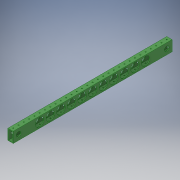
# Autodesk Inventor part: Kermit Frame 14
Saved by Autodesk Inventor 2018.2 (Build 222227000, 227)
## iProperties
Created: 2018-02-17
Part Number: Kermit Frame 14
Material: Generic
Document SubType Name: Modeling
Designer: lopez.xavier
Density: 1 g/cm^3
Appearance: Smooth - Dark Forest Green
Author: lopez.xavier
Autodesk Inventor part; units mm, degrees
ref_plane "YZ Plane" through (0, 0, 0) normal (1, 0, 0) x (0, 1, 0)
ref_plane "XZ Plane" through (0, 0, 0) normal (0, 1, 0) x (-1, 0, 0)
ref_plane "XY Plane" through (0, 0, 0) normal (0, 0, 1) x (1, 0, 0)
sketch "Sketch1" plane through (0, 0, 0) normal (0, 0, 1) x (1, 0, 0)
  line L0 (0, 0) -> (25.4, 0)
  line L1 (25.4, 0) -> (25.4, 50.8)
  line L2 (25.4, 50.8) -> (0, 50.8)
  line L3 (0, 50.8) -> (0, 0)
  dimension "d0" = 50.8
  dimension "d1" = 25.4
  constraints: 8 end point, 2 parallel, 1 horizontal, 1 perpendicular
  measures "d0" distance of L0.end L1.end
  measures "d1" distance of L1.end L2.end
extrude "Extrusion1" add sketch "Sketch1" along normal blind 762
shell "Shell1" thickness 3.175 removed faces 2 at (16.9333, 16.9333, 0) at (16.9333, 16.9333, 762)
sketch "Sketch2" plane through (25.4, 0, 0) normal (1, 0, 0) x (0, 0, -1)
  circle A0 centre (-635, 25.4) radius 20.32
  line L0 (0, 50.8) -> (-762, 50.8) projected
  circle A1 centre (-584.2, 25.4) radius 20.32
  circle A2 centre (-533.4, 25.4) radius 20.32
  circle A3 centre (-482.6, 25.4) radius 20.32
  circle A4 centre (-431.8, 25.4) radius 20.32
  circle A5 centre (-381, 25.4) radius 20.32
  circle A6 centre (-330.2, 25.4) radius 20.32
  circle A7 centre (-279.4, 25.4) radius 20.32
  circle A8 centre (-228.6, 25.4) radius 20.32
  circle A9 centre (-177.8, 25.4) radius 20.32
  circle A10 centre (-127, 25.4) radius 20.32
  line L1 (-762, 0) -> (-762, 50.8) projected
  circle A11 centre (-736.6, 25.4) radius 11.43
  circle A12 centre (-25.4, 25.4) radius 11.43
  line L2 (0, 0) -> (0, 50.8) projected
  dimension "d5" = 40.64
  dimension "d6" = 25.4
  dimension "d9" = 50.8
  dimension "d14" = 127
  dimension "d17" = 22.86
  dimension "d18" = 22.86
  dimension "d19" = 25.4
  dimension "d20" = 25.4
  dimension "d21" = 25.4
  dimension "d22" = 25.4
  constraints: 13 centre point, 1 horizontal, 20 other
  measures "d5" diameter of A0
  measures "d6" distance from line of L0 A0.centre
  measures "d9" distance of A0.centre A1.centre
  measures "d14" distance from line of L1 A0.centre
  measures "d17" diameter of A11
  measures "d18" diameter of A12
  measures "d19" distance from line of L0 A11.centre
  measures "d20" distance from line of L0 A12.centre
  measures "d21" distance from line of L1 A11.centre
  measures "d22" distance from line of L2 A12.centre
extrude "Extrusion2" cut sketch "Sketch2" against normal blind 25.4
sketch "Sketch3" plane through (0, 50.8, 0) normal (0, 1, 0) x (1, 0, 0)
  circle A0 centre (12.7, -749.3) radius 2.54
  line L0 (0, 0) -> (0, -762) projected
  line L1 (25.4, -762) -> (0, -762) projected
  circle A1 centre (12.7, -723.9) radius 2.54
  circle A2 centre (12.7, -698.5) radius 2.54
  circle A3 centre (12.7, -673.1) radius 2.54
  circle A4 centre (12.7, -647.7) radius 2.54
  circle A5 centre (12.7, -622.3) radius 2.54
  circle A6 centre (12.7, -596.9) radius 2.54
  circle A7 centre (12.7, -571.5) radius 2.54
  circle A8 centre (12.7, -546.1) radius 2.54
  circle A9 centre (12.7, -520.7) radius 2.54
  circle A10 centre (12.7, -495.3) radius 2.54
  circle A11 centre (12.7, -469.9) radius 2.54
  circle A12 centre (12.7, -444.5) radius 2.54
  circle A13 centre (12.7, -419.1) radius 2.54
  circle A14 centre (12.7, -393.7) radius 2.54
  circle A15 centre (12.7, -368.3) radius 2.54
  circle A16 centre (12.7, -342.9) radius 2.54
  circle A17 centre (12.7, -317.5) radius 2.54
  circle A18 centre (12.7, -292.1) radius 2.54
  circle A19 centre (12.7, -266.7) radius 2.54
  circle A20 centre (12.7, -241.3) radius 2.54
  circle A21 centre (12.7, -215.9) radius 2.54
  circle A22 centre (12.7, -190.5) radius 2.54
  circle A23 centre (12.7, -165.1) radius 2.54
  circle A24 centre (12.7, -139.7) radius 2.54
  circle A25 centre (12.7, -114.3) radius 2.54
  circle A26 centre (12.7, -88.9) radius 2.54
  circle A27 centre (12.7, -63.5) radius 2.54
  circle A28 centre (12.7, -38.1) radius 2.54
  circle A29 centre (12.7, -12.7) radius 2.54
  dimension "d23" = 5.08
  dimension "d24" = 12.7
  dimension "d25" = 12.7
  dimension "d28" = 25.4
  constraints: 30 centre point, 1 vertical, 58 other
  measures "d23" diameter of A0
  measures "d24" distance from line of L0 A0.centre
  measures "d25" distance from line of L1 A0.centre
  measures "d28" distance of A0.centre A1.centre
extrude "Extrusion3" cut sketch "Sketch3" against normal blind 50.8
equation "\"d20\" = d19"
body "Solid1"
